Autodesk Inventor part; units mm, degrees
(part 2 of 2)
  spline S159 degree 2 poles (30.1285, -81.8356) (30.1285, -83.2435) (28.5106, -84.9231) (27.0533, -84.9231) knots 0 0 0 1 2 2 2
  spline S160 degree 2 poles (27.0533, -84.9231) (25.738, -84.9231) (24.4042, -83.4967) (24.4042, -82.1752) knots 0 0 0 1 2 2 2
  line L114 (24.4042, -82.1752) -> (24.4042, -81.5268)
  line L115 (24.4042, -81.5268) -> (28.3377, -81.5268)
  spline S161 degree 2 poles (28.3377, -81.5268) (28.313, -81.1255) (28.0228, -80.5944) (27.7881, -80.4339) knots 0 0 0 1 2 2 2
  spline S162 degree 2 poles (27.7881, -80.4339) (27.5597, -80.2733) (26.9422, -80.1374) (26.5778, -80.1374) knots 0 0 0 1 2 2 2
  spline S163 degree 2 poles (26.5778, -80.1374) (26.2691, -80.1374) (25.6639, -80.2733) (25.4108, -80.3906) knots 0 0 0 1 2 2 2
  spline S164 degree 2 poles (25.4108, -80.3906) (25.1885, -80.4833) (24.8179, -80.7117) (24.7006, -80.7982) knots 0 0 0 1 2 2 2
  line L116 (24.7006, -80.7982) -> (24.5092, -80.7982)
  line L117 (24.5092, -80.7982) -> (24.5092, -79.3162)
  spline S165 degree 2 poles (24.5092, -79.3162) (24.7315, -79.2297) (25.0896, -79.0815) (25.4108, -79.0074) knots 0 0 0 1 2 2 2
  spline S166 degree 2 poles (25.4108, -79.0074) (25.701, -78.9271) (26.3185, -78.8407) (26.7631, -78.8407) knots 0 0 0 1 2 2 2
  spline S167 degree 2 poles (26.1703, -82.6075) (26.1826, -83.1756) (26.6828, -83.7745) (27.1953, -83.7745) knots 0 0 0 1 2 2 2
  spline S168 degree 2 poles (27.1953, -83.7745) (27.7202, -83.7745) (28.313, -83.1447) (28.3439, -82.6075) knots 0 0 0 1 2 2 2
  line L118 (28.3439, -82.6075) -> (26.1703, -82.6075)
  line L119 (55.5233, -74.0379) -> (58.1416, -66.4179)
  line L120 (58.1416, -66.4179) -> (60.1361, -66.4179)
  line L121 (60.1361, -66.4179) -> (62.7543, -74.0379)
  line L122 (62.7543, -74.0379) -> (60.7721, -74.0379)
  line L123 (60.7721, -74.0379) -> (59.111, -68.8694)
  line L124 (59.111, -68.8694) -> (57.4561, -74.0379)
  line L125 (57.4561, -74.0379) -> (55.5233, -74.0379)
  spline S169 degree 2 poles (49.1692, -70.2279) (49.1692, -69.2399) (49.4841, -67.7579) (49.8361, -67.2577) knots 0 0 0 1 2 2 2
  spline S170 degree 2 poles (49.8361, -67.2577) (50.1819, -66.7637) (51.2996, -66.2573) (52.1024, -66.2573) knots 0 0 0 1 2 2 2
  spline S171 degree 2 poles (52.1024, -66.2573) (52.9113, -66.2573) (54.0228, -66.7637) (54.3748, -67.27) knots 0 0 0 1 2 2 2
  spline S172 degree 2 poles (54.3748, -67.27) (54.7268, -67.7702) (55.0417, -69.2399) (55.0417, -70.2279) knots 0 0 0 1 2 2 2
  spline S173 degree 2 poles (55.0417, -70.2279) (55.0417, -71.2406) (54.7268, -72.6732) (54.3686, -73.1919) knots 0 0 0 1 2 2 2
  spline S174 degree 2 poles (54.3686, -73.1919) (54.0105, -73.6983) (52.8804, -74.1923) (52.1024, -74.1923) knots 0 0 0 1 2 2 2
  spline S175 degree 2 poles (52.1024, -74.1923) (51.2811, -74.1923) (50.1819, -73.6736) (49.8299, -73.161) knots 0 0 0 1 2 2 2
  spline S176 degree 2 poles (49.8299, -73.161) (49.4841, -72.6608) (49.1692, -71.185) (49.1692, -70.2279) knots 0 0 0 1 2 2 2
  spline S177 degree 2 poles (51.0897, -70.2279) (51.0897, -71.642) (51.5528, -72.7844) (52.1024, -72.7844) knots 0 0 0 1 2 2 2
  spline S178 degree 2 poles (52.1024, -72.7844) (52.6519, -72.7844) (53.1212, -71.642) (53.1212, -70.2217) knots 0 0 0 1 2 2 2
  spline S179 degree 2 poles (53.1212, -70.2217) (53.1212, -68.8261) (52.6519, -67.6652) (52.1024, -67.6652) knots 0 0 0 1 2 2 2
  spline S180 degree 2 poles (52.1024, -67.6652) (51.559, -67.6652) (51.0897, -68.8261) (51.0897, -70.2279) knots 0 0 0 1 2 2 2
  line L126 (42.3026, -68.1963) -> (43.3338, -68.1963)
  line L127 (43.3338, -68.1963) -> (43.3338, -66.3994)
  line L128 (43.3338, -66.3994) -> (45.1801, -66.3994)
  line L129 (45.1801, -66.3994) -> (45.1801, -68.1963)
  line L130 (45.1801, -68.1963) -> (48.5394, -68.1963)
  line L131 (48.5394, -68.1963) -> (48.5394, -69.6166)
  line L132 (48.5394, -69.6166) -> (45.2419, -74.0379)
  line L133 (45.2419, -74.0379) -> (43.3338, -74.0379)
  line L134 (43.3338, -74.0379) -> (43.3338, -69.5672)
  line L135 (43.3338, -69.5672) -> (42.3026, -69.5672)
  line L136 (42.3026, -69.5672) -> (42.3026, -68.1963)
  line L137 (45.1801, -69.5672) -> (45.1801, -72.1607)
  line L138 (45.1801, -72.1607) -> (47.1129, -69.5672)
  line L139 (47.1129, -69.5672) -> (45.1801, -69.5672)
  point P0 (52.4636, -6.35)
  constraints: 2 end point, 2 midpoint, 1 horizontal
extrude "Name and Version Number" cut sketch "Sketch15" against normal blind 3.175
equation "\"d14\" = gapBetweenParts"
equation "\"d16\" = gapBetweenParts"
equation "\"d18\" = gapBetweenParts"
equation "\"d20\" = gapBetweenParts"
equation "\"d21\" = gapBetweenParts"
equation "\"gapBetweenParts\" = 6.35"
body "Solid3"
